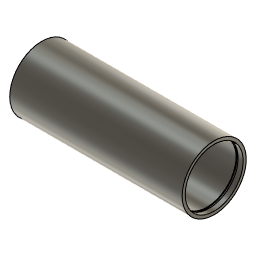
motor_case v1 (Autodesk Fusion 360 design; units mm, degrees)
Autodesk Fusion 360 part; units mm, degrees
sketch "Sketch1" plane through (0, 0, 0) normal (1, 0, 0) x (0, 1, 0)
  circle A0 centre (0, 0) radius 28.6
  circle A1 centre (0, 0) radius 31.6
  dimension "d9" = 57.2
  dimension "d10" = 63.2
  constraint coincident A0.centre A1.centre
  measures "d9" diameter of A0
  measures "d10" diameter of A1
extrude "Extrude1" add sketch "Sketch1" along normal blind 170
ref_plane "WorkPlane1" through (5, 0, 0) normal (1, 0, 0) x (0, 1, 0)
sketch "Sketch2" plane through (5, 0, 0) normal (1, 0, 0) x (0, 1, 0)
  circle A0 centre (0, 0) radius 29.5
  dimension "d14" = 59
  constraint coincident A0.centre origin
  measures "d14" diameter of A0
extrude "Extrude2" cut sketch "Sketch2" along normal blind 2
ref_plane "WorkPlane2" through (165, 0, 0) normal (1, 0, 0) x (0, 1, 0)
sketch "Sketch3" plane through (165, 0, 0) normal (1, 0, 0) x (0, 1, 0)
  circle A0 centre (0, 0) radius 29.5
  dimension "d18" = 59
  constraint coincident A0.centre origin
  measures "d18" diameter of A0
extrude "Extrude3" cut sketch "Sketch3" against normal blind 2
sketch "Sketch4" plane through (0, 0, 0) normal (1, 0, 0) x (0, 1, 0)
ref_plane "WorkPlane4" through (0, 0, 0) normal (1, 0, 0) x (0, 1, 0)
ref_plane "WorkPlane5" through (10, 0, 0) normal (1, 0, 0) x (0, 1, 0)
sketch "Sketch5" plane through (10, 0, 0) normal (1, 0, 0) x (0, 1, 0)
  circle A0 centre (0, 0) radius 29.5
  dimension "d24" = 59
  constraint coincident A0.centre origin
  measures "d24" diameter of A0
extrude "Extrude4" cut sketch "Sketch5" along normal blind 2
ref_plane "WorkPlane6" through (14, 0, 0) normal (1, 0, 0) x (0, 1, 0)
sketch "Sketch6" plane through (14, 0, 0) normal (1, 0, 0) x (0, 1, 0)
  circle A0 centre (0, 0) radius 29.5
  dimension "d28" = 59
  constraint coincident A0.centre origin
  measures "d28" diameter of A0
extrude "Extrude5" cut sketch "Sketch6" along normal blind 2
